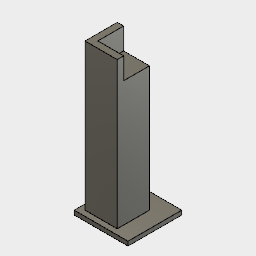
60mm柱 v1 (Autodesk Fusion 360 design; units mm, degrees)
Autodesk Fusion 360 part; units mm, degrees
sketch "スケッチ1" plane through (0, 0, 0) normal (0, 1, 0) x (1, 0, 0)
  line L0 (10, -10) -> (-10, -10)
  line L1 (-10, -10) -> (-10, 10)
  line L2 (-10, 10) -> (10, 10)
  line L3 (10, 10) -> (10, -10)
  line L4 (10, -10) -> (-10, 10) construction
  line L5 (-10, -10) -> (10, 10) construction
  dimension "d1" = 20
  dimension "d2" = 20
  measures "d1" distance of L1.end L2.end
  measures "d2" distance of L0.end L1.end
extrude "押し出し1" add sketch "スケッチ1" along normal blind 2
sketch "スケッチ2" plane through (0, 2, 0) normal (0, 1, 0) x (-1, 0, 0)
  line L0 (-10, -10) -> (10, -10)
  line L1 (10, -10) -> (10, 10)
  line L2 (10, 10) -> (-10, 10)
  line L3 (-10, 10) -> (-10, -10)
  line L4 (-7.5, 7.5) -> (7.5, 7.5)
  line L5 (7.5, 7.5) -> (7.5, -7.5)
  line L6 (7.5, -7.5) -> (-7.5, -7.5)
  line L7 (-7.5, -7.5) -> (-7.5, 7.5)
  line L8 (-7.5, 7.5) -> (7.5, -7.5) construction
  line L9 (7.5, 7.5) -> (-7.5, -7.5) construction
  dimension "d5" = 15
  dimension "d6" = 15
  measures "d5" distance of L4.end L5.end
  measures "d6" distance of L5.end L6.end
extrude "押し出し2" add sketch "スケッチ2" along normal blind 58 contours L4 L5 L6 L7
sketch "スケッチ3" plane through (0, 60, 0) normal (0, 1, 0) x (-1, 0, 0)
  line L0 (-7.5, -7.5) -> (7.5, -7.5)
  line L1 (7.5, -7.5) -> (7.5, 7.5)
  line L2 (7.5, 7.5) -> (-7.5, 7.5)
  line L3 (-7.5, 7.5) -> (-7.5, -7.5)
  line L4 (4.5, -7.5) -> (4.5, 4.5)
  line L5 (4.5, 4.5) -> (-7.5, 4.5)
  dimension "d9" = 3
  dimension "d10" = 3
  measures "d9" distance of L1 L4
  measures "d10" distance of L2 L5
extrude "押し出し3" add sketch "スケッチ3" along normal blind 10 contours L0 L1 L2 L3 L4 L5
move_face "面をオフセット1" offset 5 1 faces at (10, 0.6667, -3.3333)
move_face "面をオフセット2" offset 5 1 faces at (6.6667, 1.3333, -10)
